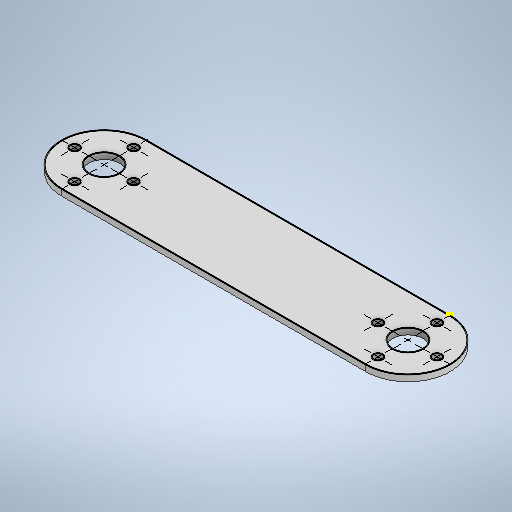
# Autodesk Inventor part: CAM_axis_4_5_connector_frame_non_powered
Saved by Autodesk Inventor 2025.2 (Build 292293000, 293)
## iProperties
Created: 2025-08-09
Part Number: CAM_axis_4_5_connector_frame_non_powered
Material: Generic
Document SubType Name: Modeling
Designer: User
Density: 1 g/cm^3
Appearance: Default
Author: User
Autodesk Inventor part; units mm, degrees
ref_plane "YZ Plane" through (0, 0, 0) normal (1, 0, 0) x (0, 1, 0)
ref_plane "XZ Plane" through (0, 0, 0) normal (0, 1, 0) x (-1, 0, 0)
ref_plane "XY Plane" through (0, 0, 0) normal (0, 0, 1) x (1, 0, 0)
sketch "Sketch1" plane through (0, 0, 0) normal (0, 1, 0) x (-1, 0, 0)
  circle A0 centre (72.1, 10) radius 3.6
  circle A1 centre (0, 10) radius 3.6
  circle A2 centre (7.1, 10) radius 1.05
  circle A3 centre (0.1, 3) radius 1.05
  circle A4 centre (-6.9, 10) radius 1.05
  circle A5 centre (0.1, 17) radius 1.05
  circle A6 centre (65.1, 10) radius 1.05
  circle A7 centre (79.1, 10) radius 1.05
  circle A8 centre (72.1, 17) radius 1.05
  circle A9 centre (72.1, 3) radius 1.05
  arc A10 (0, 20) -> (0, 0) centre (0, 10) ccw
  arc A11 (72.1, 0) -> (72.1, 20) centre (72.1, 10) ccw
  line L0 (72.1, 0) -> (0, 0)
  line L1 (0, 20) -> (72.1, 20)
  point P0 (0, 0)
  constraints: 12 centre point, 9 equal radius, 4 end point, 4 point on circle, 4 tangent, 2 horizontal, 27 other
extrude "Extrusion1" add sketch "Sketch1" against normal blind 1.5
body "Solid1"
